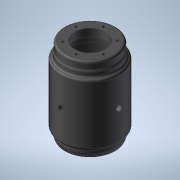
# Autodesk Inventor part: inside
Saved by Autodesk Inventor 2020.2 (Build 242310000, 310)
## iProperties
Created: 2019-07-19
Part Number: inside
Material: Generic
Document SubType Name: Modeling
Designer: njk024
Density: 1 g/cm^3
Appearance: Default
Author: njk024
Autodesk Inventor part; units mm, degrees
ref_plane "XZ Plane" through (0, 0, 0) normal (0, 1, 0) x (-1, 0, 0)
sketch "Sketch2" plane through (0, 0, 0) normal (0, 0, 1) x (1, 0, 0)
  line L0 (111.0613, -64.0334) -> (111.0613, -182.5498) construction
  arc A0 (111.0613, -182.5498) -> (111.0613, -64.0334) centre (111.0613, -123.2916) ccw construction
  line L1 (170.3195, -123.2916) -> (170.3195, -29.6291) construction
  line L2 (170.3195, -29.6291) -> (170.3195, -216.9541) construction
  line L3 (111.0613, -64.0334) -> (106.2861, -64.0334) construction
  line L4 (111.0613, -182.5498) -> (106.2861, -182.5498) construction
  line L5 (106.2861, -64.0334) -> (106.2861, -70.3834) construction
  line L6 (60.2613, -34.4043) -> (60.2613, -212.1789) construction
  line L7 (106.2861, -182.5498) -> (106.2861, -176.1998) construction
  line L8 (106.2861, -70.3834) -> (111.0613, -70.3834) construction
  line L9 (111.0613, -70.3834) -> (111.0613, -176.1998) construction
  line L10 (106.2861, -176.1998) -> (111.0613, -176.1998) construction
  line L11 (111.0613, -64.0334) -> (138.1631, -64.0334) construction
  line L12 (111.0613, -182.5498) -> (138.1631, -182.5498) construction
  arc A1 (138.1631, -182.5498) -> (138.1631, -64.0334) centre (108.1245, -123.2916) ccw construction
  line L13 (174.5613, -123.2916) -> (174.5613, -216.9541) construction
  line L14 (104.2861, -72.3834) -> (104.2861, -62.0334)
  line L15 (104.2861, -62.0334) -> (103.0161, -62.0334)
  line L16 (104.2861, -72.3834) -> (109.0613, -72.3834)
  line L17 (109.0613, -72.3834) -> (109.0613, -123.2916)
  line L18 (109.0613, -123.2916) -> (174.5613, -123.2916) construction
  line L19 (104.2861, -174.1998) -> (104.2861, -184.5498)
  line L20 (104.2861, -184.5498) -> (103.0161, -184.5498)
  line L21 (104.2861, -174.1998) -> (109.0613, -174.1998)
  line L22 (109.0613, -174.1998) -> (109.0613, -123.2916)
  line L23 (103.0161, -62.0334) -> (103.0161, -49.3334)
  line L24 (103.0161, -49.3334) -> (97.9361, -49.3334)
  line L25 (97.9361, -49.3334) -> (97.9361, -78.7334)
  line L26 (97.9361, -78.7334) -> (102.7113, -78.7334)
  line L27 (102.7113, -78.7334) -> (102.7113, -167.8498)
  line L28 (102.7113, -167.8498) -> (95.1523, -167.8498)
  line L29 (95.1523, -189.6298) -> (103.0161, -189.6298)
  line L30 (103.0161, -189.6298) -> (103.0161, -184.5498)
  line L31 (95.1523, -167.8498) -> (60.2613, -167.8498)
  line L32 (95.1523, -189.6298) -> (60.2613, -189.6298)
  line L33 (60.2613, -167.8498) -> (60.2613, -189.6298)
  point P0 (0, 0)
  dimension "d0" = 59.2582
  dimension "d1" = 59.2582
  dimension "d2" = 4.7752
  dimension "d3" = 4.7752
  dimension "d4" = 6.35
  dimension "d5" = 50.8
  dimension "d7" = 27.1018
  dimension "d8" = 114.3
  dimension "d9" = 27.1018
  dimension "d10" = 105.8164
  dimension "d12" = 2
  dimension "d13" = 2
  dimension "d14" = 2
  dimension "d15" = 2
  dimension "d16" = 12.7
  dimension "d17" = 6.35
  dimension "d18" = 6.35
  dimension "d19" = 6.35
  dimension "d20" = 6.35
  dimension "d21" = 5.08
  dimension "d35" = 5.08
  constraints: 68 end point, 11 perpendicular, 7 vertical, 6 point on circle, 5 horizontal, 5 point on line, 4 symmetric about line, 4 tangent, 2 centre point, 2 parallel, 1 collinear, 1 midpoint
  measures "d0" radius of A0
  measures "d1" distance between parallel lines of L1 L0
  measures "d2" distance of L11.start L3.end
  measures "d3" distance of L0.end L4.end
  measures "d4" distance of L3.end L5.end
  measures "d5" distance between parallel lines of L0 L6
  measures "d7" distance of L0.end L12.end
  measures "d8" distance between parallel lines of L6 L13
  measures "d9" distance of L11.start L11.end
  measures "d10" distance of L9.start L9.end
  measures "d12" distance between parallel lines of L5 L14
  measures "d13" distance between parallel lines of L15 L3
  measures "d14" distance between parallel lines of L16 L8
  measures "d15" distance between parallel lines of L0 L17
  measures "d16" distance of L15.end L23.end
  measures "d17" distance between parallel lines of L14 L25
  measures "d18" distance between parallel lines of L26 L16
  measures "d19" distance between parallel lines of L17 L27
  measures "d20" distance between parallel lines of L21 L28
  measures "d21" distance between parallel lines of L29 L20
  measures "d35" distance of L23.end L24.end
revolve "Revolution2" add sketch "Sketch2" angle 360 about axis through (60.2613, -34.4043, 0) along (0, -1, 0)
fillet "Fillet1" radius 3.175 1 edges at (16.2365, -72.3834, 0)
fillet "Fillet2" radius 3.175 1 edges at (16.2365, -62.0334, 0)
fillet "Fillet3" radius 3.175 1 edges at (16.2365, -174.1998, 0)
fillet "Fillet4" radius 3.175 1 edges at (16.2365, -184.5498, 0)
fillet "Fillet5" radius 3.175 1 edges at (11.4613, -72.3834, 0)
fillet "Fillet6" radius 3.175 1 edges at (11.4613, -174.1998, 0)
fillet "Fillet7" radius 3.175 1 edges at (17.5065, -49.3334, 0)
fillet "Fillet8" radius 3.175 1 edges at (17.5065, -62.0334, 0)
fillet "Fillet9" radius 3.175 1 edges at (17.5065, -184.5498, 0)
fillet "Fillet10" radius 3.175 1 edges at (17.5065, -189.6298, 0)
ref_plane "Work Plane2" through (0, 0, 65.0875) normal (0, 0, 1) x (1, 0, 0)
sketch "Sketch3" plane through (0, 0, 65.0875) normal (0, 0, 1) x (1, 0, 0)
  line L0 (109.0613, -75.36) -> (11.4613, -75.36) construction
  line L1 (11.4613, -171.2232) -> (109.0613, -171.2232) construction
  line L2 (11.4613, -75.36) -> (11.4613, -171.2232) construction
  line L3 (109.0613, -171.2232) -> (109.0613, -75.36) construction
  line L4 (106.6737, -174.299) -> (13.8489, -174.299) construction
  line L5 (11.4613, -123.2916) -> (109.0613, -123.2916) construction
  line L6 (60.2613, -75.36) -> (60.2613, -171.2232) construction
  circle A0 centre (60.2613, -123.2916) radius 4.9022
  point P0 (0, 0)
  dimension "d37" = 9.8044
  constraints: 8 end point, 5 midpoint, 1 centre point, 1 perpendicular, 1 vertical
  measures "d37" diameter of A0
extrude "Extrusion1" cut sketch "Sketch3" against normal through all
ref_plane "Work Plane3" through (-20.6375, 0, 0) normal (1, 0, 0) x (0, 1, 0)
sketch "Sketch4" plane through (-20.6375, 0, 0) normal (1, 0, 0) x (0, 1, 0)
  line L0 (-75.36, -48.8) -> (-75.36, 48.8) construction
  line L1 (-171.2232, 48.8) -> (-171.2232, -48.8) construction
  line L2 (-75.36, -48.8) -> (-171.2232, -48.8) construction
  line L3 (-75.36, 48.8) -> (-171.2232, 48.8) construction
  line L4 (-123.2916, -48.8) -> (-123.2916, 48.8) construction
  line L5 (-75.36, 0) -> (-171.2232, 0) construction
  circle A0 centre (-123.2916, 0) radius 4.9022
  point P0 (0, 0)
  dimension "d41" = 9.8044
  constraints: 8 end point, 5 midpoint, 2 horizontal, 1 centre point
  measures "d41" diameter of A0
extrude "Extrusion2" cut sketch "Sketch4" along normal blind 188.4364
sketch "Sketch5" plane through (60.2613, -49.3334, 0) normal (0, 1, 0) x (1, 0, 0)
  circle A0 centre (0, 0) radius 39.5798 projected
  point P0 (-60.2613, 0)
extrude "Extrusion3" add sketch "Sketch5" against normal blind 12.7
sketch "Sketch6" plane through (60.2613, -49.3334, 0) normal (0, 1, 0) x (1, 0, 0)
  circle A0 centre (0, 0) radius 25.4
  point P0 (-60.2613, 0)
  dimension "d46" = 50.8
  constraints: 1 centre point
  measures "d46" diameter of A0
extrude "Extrusion4" cut sketch "Sketch6" against normal blind 12.7
sketch "Sketch7" plane through (60.2613, -189.6298, 0) normal (0, -1, 0) x (1, 0, 0)
  circle A0 centre (0, 0) radius 39.5798 construction
  line L0 (-39.5798, 0) -> (39.5798, 0) construction
  line L1 (0, -39.5798) -> (0, 39.5798) construction
  circle A1 centre (0, 0) radius 39.5798 construction
  line L2 (0, 0) -> (19.7899, -34.2771) construction
  line L3 (0, 0) -> (19.7899, 34.2771) construction
  line L4 (0, 0) -> (-39.5798, 0) construction
  circle A2 centre (0, 0) radius 19.7899 construction
  circle A3 centre (0, 0) radius 28.575 construction
  circle A4 centre (0, 0) radius 42.45 projected
  circle A5 centre (0, 0) radius 17
  point P0 (-60.2613, 0)
  dimension "d51" = 120
  dimension "d53" = 120
  dimension "d54" = 120
  dimension "d55" = 79.1596
  dimension "d56" = 39.5798
  dimension "d58" = 57.15
  dimension "d59" = 34
  constraints: 10 end point, 4 point on circle, 3 centre point, 3 coincident, 1 horizontal, 1 vertical, 4 other
  measures "d51" angle of L0 L2
  measures "d53" angle of L3 L2
  measures "d54" angle of L4 L3
  measures "d55" diameter of A0
  measures "d56" diameter of A2
  measures "d58" diameter of A3
  measures "d59" diameter of A5
extrude "Extrusion5" cut sketch "Sketch7" against normal up to next contours A5
sketch "Sketch11" plane through (60.2613, -49.3334, 0) normal (0, 1, 0) x (1, 0, 0)
  circle A0 centre (-20.8699, -24.8718) radius 2.1
  circle A1 centre (0, 0) radius 39.5798 construction
  line L0 (-25.8988, -29.9007) -> (-15.8722, -19.8741) construction
  circle A2 centre (0, 0) radius 25.4 construction
  line L1 (-25.8988, -29.9007) -> (-47.8914, -7.9082) construction
  circle A3 centre (0, 0) radius 39.5798 construction
  circle A4 centre (8.4033, -31.3615) radius 2.1
  circle A5 centre (31.3615, -8.4033) radius 2.1
  circle A6 centre (22.9582, 22.9582) radius 2.1
  circle A7 centre (-8.4033, 31.3615) radius 2.1
  circle A8 centre (-31.3615, 8.4033) radius 2.1
  point P0 (-60.2613, 0)
  dimension "d78" = 4.2
  dimension "d79" = 14.1798
  dimension "d81" = 7.112
  dimension "d84" = 360
  constraints: 6 centre point, 4 end point, 2 other
  measures "d78" diameter of A0
  measures "d79" radial gap between concentric circles of A2 A1
  measures "d81" distance from line of A0.centre L1
extrude "M4 mounting holes" cut sketch "Sketch11" against normal up to next
sketch "Sketch16" plane through (60.2613, -189.6298, 0) normal (0, -1, 0) x (1, 0, 0)
  line L0 (0, 42.634) -> (0, -47.7883) construction
  line L1 (-45.263, 0) -> (45.3317, 0) construction
  circle A0 centre (0, 30.48) radius 3.5052
  line L2 (0, 30.48) -> (0.0344, 0) construction
  circle A1 centre (-30.4456, -0.0344) radius 3.5052
  circle A2 centre (0.0687, -30.48) radius 3.5052
  circle A3 centre (30.5144, 0.0344) radius 3.5052
  point P0 (-60.2613, 0)
  dimension "d109" = 7.0104
  dimension "d110" = 30.48
  dimension "d113" = 360
  constraints: 6 end point, 4 centre point, 2 horizontal, 1 midpoint, 1 point on line, 1 vertical, 9 other
  measures "d109" diameter of A0
  measures "d110" distance from line of L2.start L1
extrude "Extrusion14" cut sketch "Sketch16" against normal up to next
sketch "Sketch21" plane through (60.2613, -189.6298, 0) normal (0, -1, 0) x (1, 0, 0)
  circle A0 centre (0, 0) radius 39.5798 construction
  line L0 (39.5798, 0) -> (-39.5798, 0) construction
  line L1 (0, 39.5798) -> (0, -39.5798) construction
  circle A1 centre (30.5144, 0.0344) radius 3.5052 construction
  circle A2 centre (0, 30.48) radius 3.5052 construction
  circle A3 centre (-30.4456, -0.0344) radius 3.5052 construction
  circle A4 centre (0.0687, -30.48) radius 3.5052 construction
  circle A5 centre (0, 0) radius 30.4801 construction
  circle A6 centre (-21.5527, 21.5527) radius 3.5
  circle A7 centre (0, 0) radius 42.45 construction
  line L2 (-21.5527, 21.5527) -> (0, 0) construction
  circle A8 centre (0, 0) radius 25.4 construction
  line L3 (0, 0) -> (21.5527, -21.5527) construction
  circle A9 centre (21.5527, -21.5527) radius 3.5
  point P0 (-60.2613, 0)
  dimension "d139" = 7
  dimension "d140" = 135
  dimension "d141" = 7
  dimension "d149" = 45
  constraints: 8 end point, 7 point on circle, 3 centre point, 2 coincident, 1 horizontal, 1 vertical
  measures "d139" diameter of A6
  measures "d140" angle of L0 L2
  measures "d141" diameter of A9
  measures "d149" angle of L0 L3
extrude "Extrusion17" cut sketch "Sketch21" against normal up to next
sketch "Sketch22" plane through (60.2613, -189.6298, 0) normal (0, -1, 0) x (1, 0, 0)
  circle A0 centre (-21.5527, 21.5527) radius 3.5 projected
  circle A1 centre (21.5527, -21.5527) radius 3.5 projected
  circle A2 centre (-21.5527, 21.5527) radius 5.08
  circle A3 centre (21.5527, -21.5527) radius 3.5 construction
  circle A4 centre (21.5527, -21.5527) radius 5.08
  point P0 (-60.2613, 0)
  dimension "d144" = 10.16
  dimension "d145" = 10.16
  constraints: 2 centre point, 2 coincident
  measures "d144" diameter of A2
  measures "d145" diameter of A4
extrude "Extrusion18" add sketch "Sketch22" along normal blind 3
fillet "Fillet12" radius 3.175 2 edges at (33.6287, -189.6298, 21.5527) (76.734, -189.6298, -21.5527)
equation "\"d56\" = 0.5 * d55"
body "Solid2"
